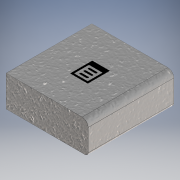
# Autodesk Inventor part: PRZYCISK IO
Saved by Autodesk Inventor 2017 SP1 (Build 210196100, 196)
## iProperties
Created: 2021-03-07
Part Number: PRZYCISK IO
Material: Tworzywo sztuczne, nieprzezroczyste czarne
Document SubType Name: Modeling
Designer: Administrator
Density: 0.952 g/cm^3
Appearance: Teksturowany - szary
Author: Administrator
Autodesk Inventor part; units mm, degrees
ref_plane "YZ Plane" through (0, 0, 0) normal (1, 0, 0) x (0, 1, 0)
ref_plane "XZ Plane" through (0, 0, 0) normal (0, 1, 0) x (-1, 0, 0)
ref_plane "XY Plane" through (0, 0, 0) normal (0, 0, 1) x (1, 0, 0)
sketch "Szkic1" plane through (0, 0, 0) normal (0, 0, 1) x (1, 0, 0)
  line L0 (206.45, -143.65) -> (206.45, -129.275)
  line L1 (206.45, -129.275) -> (220.2, -129.275)
  line L2 (206.45, -143.65) -> (220.2, -143.65)
  line L3 (220.2, -129.275) -> (220.2, -143.65)
  constraints: 8 end point
extrude "Wyciągnięcie proste1" add sketch "Szkic1" against normal blind 5.2
fillet "Zaokrąglenie1" radius 0.5 1 edges at (220.2, -136.4625, -5.2)
fillet "Zaokrąglenie2" radius 1 1 edges at (220.2, -136.4625, 0)
sketch "Szkic6" plane through (0, 0, 0) normal (0, 0, 1) x (1, 0, 0)
  line L0 (211.8933, -134.5998) -> (214.7567, -134.5998)
  line L1 (214.8067, -134.6498) -> (214.8067, -138.2752)
  line L2 (214.7567, -138.3252) -> (211.8933, -138.3252)
  line L3 (211.8433, -138.2752) -> (211.8433, -134.6498)
  line L4 (212.2433, -137.9752) -> (214.4067, -137.9752)
  line L5 (214.4567, -137.9252) -> (214.4567, -135.5548)
  line L6 (212.1933, -135.5548) -> (212.1933, -137.9252)
  line L7 (214.4067, -135.5048) -> (212.2433, -135.5048)
  line L8 (212.75, -137.6248) -> (213.9, -137.6248)
  line L9 (213.9, -137.2748) -> (212.75, -137.2748)
  arc A0 (212.75, -137.2748) -> (212.75, -137.6248) centre (212.75, -137.4498) ccw
  arc A1 (213.9, -137.6248) -> (213.9, -137.2748) centre (213.9, -137.4498) ccw
  line L10 (212.75, -136.9048) -> (213.9, -136.9048)
  line L11 (213.9, -136.5548) -> (212.75, -136.5548)
  arc A2 (212.75, -136.5548) -> (212.75, -136.9048) centre (212.75, -136.7298) ccw
  arc A3 (213.9, -136.9048) -> (213.9, -136.5548) centre (213.9, -136.7298) ccw
  line L12 (212.75, -136.2048) -> (213.9, -136.2048)
  line L13 (213.9, -135.8548) -> (212.75, -135.8548)
  arc A4 (212.75, -135.8548) -> (212.75, -136.2048) centre (212.75, -136.0298) ccw
  arc A5 (213.9, -136.2048) -> (213.9, -135.8548) centre (213.9, -136.0298) ccw
  arc A6 (214.8067, -134.6498) -> (214.7567, -134.5998) centre (214.7567, -134.6498) ccw
  arc A7 (214.7567, -138.3252) -> (214.8067, -138.2752) centre (214.7567, -138.2752) ccw
  arc A8 (211.8933, -134.5998) -> (211.8433, -134.6498) centre (211.8933, -134.6498) ccw
  arc A9 (211.8433, -138.2752) -> (211.8933, -138.3252) centre (211.8933, -138.2752) ccw
  arc A10 (212.1933, -137.9252) -> (212.2433, -137.9752) centre (212.2433, -137.9252) ccw
  arc A11 (212.2433, -135.5048) -> (212.1933, -135.5548) centre (212.2433, -135.5548) ccw
  arc A12 (214.4567, -135.5548) -> (214.4067, -135.5048) centre (214.4067, -135.5548) ccw
  arc A13 (214.4067, -137.9752) -> (214.4567, -137.9252) centre (214.4067, -137.9252) ccw
  point P0 (213.325, -137.4498)
  point P1 (213.325, -136.7298)
  point P2 (213.325, -137.4498)
  point P3 (213.325, -136.7298)
  point P4 (213.325, -136.0298)
  dimension "d80" = 0.175
  constraints: 28 end point, 28 point on circle, 28 tangent, 14 centre point, 6 equal radius, 5 parallel, 2 horizontal, 2 perpendicular, 1 vertical
  measures "d80" radius of A2
extrude "Wyciągnięcie proste5" add sketch "Szkic6" along normal blind 0.001
